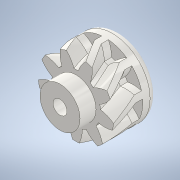
# Autodesk Inventor part: Spur Gear1
Saved by Autodesk Inventor 2022 (Build 260153070, 153G)
## iProperties
CustomPartVersion: 1
Created: 2022-01-11
Part Number: Spur Gear1
Material: Steel
Document SubType Name: Modeling
Designer: a laptop
Categories: <?xml version="1.0" encoding="UTF-16"?> <MemberInstance><Categories><FamilyTemplate><FamilyTemplateParameter ValueType="xs:double" Id="1" ObjectReferenceKey="da_z" ObjectType="kUserParameterObject"/><FamilyTemplateParameter ValueType="xs:double" Id="2" ObjectReferenceKey="da_b" ObjectType="kUserParameterObject"/><FamilyTemplateParameter ValueType="xs:double" Id="3" ObjectReferenceKey="da_beta" ObjectType="kUserParameterObject"/><FamilyTemplateParameter ValueType="xs:double" Id="4" ObjectReferenceKey="da_da" ObjectType="kUserParameterObject"/><FamilyTemplateParameter ValueType="xs:double" Id="5" ObjectReferenceKey="da_aw" ObjectType="kUserParameterObject"/><FamilyTemplateParameter ValueType="xs:string" Id="6" ObjectReferenceKey="EAIAABAAAACIAQAAAAAAAIAAAAAAAAAA" ObjectType="83910656" SubObjectId="SurfaceGeometry"/></FamilyTemplate><ParamToTemplateMap><ParamToTemplate CategoryParameter="//CategoryParameter[@InternalName='046C89C9-8512-4d59-83FE-43B91F4F132A']" TemplateParameter="1"/><ParamToTemplate CategoryParameter="//CategoryParameter[@InternalName='2552DF32-E462-4b46-AEBF-C6C7768E72AC']" TemplateParameter="2"/><ParamToTemplate CategoryParameter="//CategoryParameter[@InternalName='C9EE641D-15FC-4fae-A226-E94C4372FDD7']" TemplateParameter="3"/><ParamToTemplate><ParamToTemplate CategoryParameter="//CategoryParameter[@InternalName='00B6519A-459B-49c7-AD84-2E56D39A5744']" ConstantValue="0.510375"/></ParamToTemplate><ParamToTemplate><ParamToTemplate CategoryParameter="//CategoryParameter[@InternalName='04B31F0E-C7A6-4894-AA32-9629BEFACF47']" ConstantValue="1.000000"/></ParamToTemplate><ParamToTemplate><ParamToTemplate CategoryParameter="//CategoryParameter[@InternalName='43CBEC2E-7847-49e7-A936-2F7889FCB2D9']" ConstantValue="0.250000"/></ParamToTemplate><ParamToTemplate><ParamToTemplate CategoryParameter="//CategoryParameter[@InternalName='B1EFC894-105D-4ebd-86BF-FA20ED196853']" ConstantValue="0.302500"/></ParamToTemplate><ParamToTemplate><ParamToTemplate CategoryParameter="//CategoryParameter[@InternalName='51175063-3D10-4879-93E8-6246FE8B403D']" ConstantValue="2060000000.000000"/></ParamToTemplate><ParamToTemplate><ParamToTemplate CategoryParameter="//CategoryParameter[@InternalName='A3A52E27-4454-46a9-B0BD-C932399B70AF']" ConstantValue="0.300000"/></ParamToTemplate><ParamToTemplate><ParamToTemplate CategoryParameter="//CategoryParameter[@InternalName='91B76062-C214-41d9-B1B9-14D2AB99603D']" ConstantValue="0.080000"/></ParamToTemplate><ParamToTemplate><ParamToTemplate CategoryParameter="//CategoryParameter[@InternalName='374E806E-8B8A-4dda-A9AA-1039D6500AD2']" ConstantValue="12.500000"/></ParamToTemplate><ParamToTemplate><ParamToTemplate CategoryParameter="//CategoryParameter[@InternalName='2D373A89-B862-43d6-8D0B-0CBF12AB9F6C']" ConstantValue="0.261799"/></ParamToTemplate><ParamToTemplate CategoryParameter="//CategoryParameter[@InternalName='37777632-D6A2-4fac-9D53-DB8ACD95C989']" TemplateParameter="4"/><ParamToTemplate CategoryParameter="//CategoryParameter[@InternalName='FD1017F1-B727-4f7e-9707-0F86F1FF9423']" TemplateParameter="5"/><ParamToTemplate><ParamToTemplate CategoryParameter="//CategoryParameter[@InternalName='9E1B4470-B2D3-4ff1-B813-535BB4CDF51A']" ConstantValue="3520000.000000"/></ParamToTemplate><ParamToTemplate><ParamToTemplate CategoryParameter="//CategoryParameter[@InternalName='F8452263-BFF6-458c-9FB1-07C4B99E95CD']" ConstantValue="11400000.000000"/></ParamToTemplate><ParamToTemplate><ParamToTemplate CategoryParameter="//CategoryParameter[@InternalName='3E3BB259-FD49-497f-8171-6EBC954A3479']" ConstantValue="2.000000"/></ParamToTemplate><ParamToTemplate CategoryParameter="//CategoryParameter[@InternalName='27C3BAF2-7550-4e4b-AE2C-0DB134B7D9B7']" TemplateParameter="6"/></ParamToTemplateMap><Category DisplayName="Gear" InternalName="DC85795E-93AB-48d5-8EEE-5A27447B64BD" Mnemonic="Gear"><CategoryParameter DisplayName="z" InternalName="046C89C9-8512-4d59-83FE-43B91F4F132A" Mnemonic="z"/><CategoryParameter DisplayName="b" InternalName="2552DF32-E462-4b46-AEBF-C6C7768E72AC" Mnemonic="b"/><CategoryParameter DisplayName="||b|" InternalName="C9EE641D-15FC-4fae-A226-E94C4372FDD7" Mnemonic="beta"/><CategoryParameter DisplayName="x" InternalName="00B6519A-459B-49c7-AD84-2E56D39A5744" Mnemonic="x"/><CategoryParameter DisplayName="a*" InternalName="04B31F0E-C7A6-4894-AA32-9629BEFACF47" Mnemonic="a"/><CategoryParameter DisplayName="c*" InternalName="43CBEC2E-7847-49e7-A936-2F7889FCB2D9" Mnemonic="c"/><CategoryParameter DisplayName="r|.f|*" InternalName="B1EFC894-105D-4ebd-86BF-FA20ED196853" Mnemonic="rf"/><CategoryParameter DisplayName="E" InternalName="51175063-3D10-4879-93E8-6246FE8B403D" Mnemonic="E"/><CategoryParameter DisplayName="||m|" InternalName="A3A52E27-4454-46a9-B0BD-C932399B70AF" Mnemonic="mi"/><Category DisplayName="SpurGear" InternalName="26C5A22E-A91E-4dfd-A3B3-23CCAFAE1764" Mnemonic="SpurGear"><CategoryParameter DisplayName="m" InternalName="91B76062-C214-41d9-B1B9-14D2AB99603D" Mnemonic="m"/><CategoryParameter DisplayName="P" InternalName="374E806E-8B8A-4dda-A9AA-1039D6500AD2" Mnemonic="PP"/><CategoryParameter DisplayName="||a|" InternalName="2D373A89-B862-43d6-8D0B-0CBF12AB9F6C" Mnemonic="alpha"/><CategoryParameter DisplayName="d|.a|" InternalName="37777632-D6A2-4fac-9D53-DB8ACD95C989" Mnemonic="da"/><CategoryParameter DisplayName="a|.w|" InternalName="FD1017F1-B727-4f7e-9707-0F86F1FF9423" Mnemonic="aw"/><CategoryParameter DisplayName="||s||.Flim|" InternalName="9E1B4470-B2D3-4ff1-B813-535BB4CDF51A" Mnemonic="sFlim"/><CategoryParameter DisplayName="||s||.Hlim|" InternalName="F8452263-BFF6-458c-9FB1-07C4B99E95CD" Mnemonic="sHlim"/><CategoryParameter DisplayName="type" InternalName="3E3BB259-FD49-497f-8171-6EBC954A3479" Mnemonic="type"/><CategoryParameter DisplayName="PitchDiameter" InternalName="27C3BAF2-7550-4e4b-AE2C-0DB134B7D9B7" Mnemonic="IDS_PITCHDIAM"/></Category></Category></Categories></MemberInstance>
Mass: 1.41514 g
Surface Area: 2.76854 cm^2
Volume: 0.180272 cm^3
Density: 7.85 g/cm^3
Appearance: Steel
Author: a laptop
Autodesk Inventor part; units mm, degrees
ref_plane "YZ Plane" through (0, 0, 0) normal (1, 0, 0) x (0, 1, 0)
ref_plane "XZ Plane" through (0, 0, 0) normal (0, 1, 0) x (-1, 0, 0)
ref_plane "XY Plane" through (0, 0, 0) normal (0, 0, 1) x (1, 0, 0)
sketch "Sketch1" plane through (0, 0, 0) normal (0, 0, 1) x (1, 0, 0)
  circle A0 centre (0, 0) radius 5.1751
  dimension "d0" = 10.3501
  constraints: 1 centre point
  measures "d0" diameter of A0
extrude "Extrusion1" add sketch "Sketch1" along normal blind 3
ref_plane "Work Plane2" through (0, 0, 1.5) normal (0, 0, 1) x (1, 0, 0)
sketch "Sketch2" plane through (0, 0, 0) normal (0, 0, -1) x (-1, 0, 0)
  circle A0 centre (0, 0) radius 5.1751 projected
  circle A1 centre (0, 0) radius 3.9722
  dimension "d3" = 7.9443
  constraints: 1 centre point, 1 coincident
  measures "d3" diameter of A1
surface extrude "Pitch Diameter" sketch "Sketch2" against normal through all shown no curves A1
ref_plane "Work Plane8" through (0, 0, 0) normal (0.9396926, 0.3420201, 0) x (0, 0, 1)
ref_plane "Work Plane9" through (0, 0, 0) normal (1, 0, 0) x (0, 1, 0)
spur gear teeth "Spur Gear" teeth 9 pitch diameter 7.9443 tip diameter 10.3501 root diameter 6.7609 face width 3 helix angle 25 hand left start plane through (0, 0, 0) normal (0, 0, -1) x (-1, 0, 0)
sketch "Sketch3" plane through (0, 0, 0) normal (0, 0, -1) x (-1, 0, 0)
  spline S0 degree 6 poles (2.7691, 1.939) (2.9838, 2.1842) (3.1749, 2.4503) (3.3397, 2.7342) (3.4763, 3.0327) (3.5831, 3.3423) (3.6593, 3.6593) knots 0 0 0 0 0 0 0 1 1 1 1 1 1 1 projected
  arc A0 (3.6593, 3.6593) -> (2.9683, 4.2392) centre (0, 0) ccw projected
  spline S1 degree 6 poles (2.9683, 4.2392) (2.6694, 4.1091) (2.383, 3.9501) (2.1127, 3.7638) (1.8617, 3.5521) (1.6329, 3.3178) (1.4286, 3.0637) knots 0 0 0 0 0 0 0 1 1 1 1 1 1 1 projected
  spline S2 degree 6 poles (1.4286, 3.0637) (1.3395, 3.1053) (1.249, 3.1437) (1.1571, 3.179) (1.064, 3.2111) (0.9699, 3.2398) (0.8749, 3.2653) knots 0 0 0 0 0 0 0 1 1 1 1 1 1 1 projected
  spline S3 degree 6 poles (0.8749, 3.2653) (0.8818, 3.5912) (0.8571, 3.9178) (0.8009, 4.2412) (0.7136, 4.5577) (0.5964, 4.8636) (0.451, 5.1554) knots 0 0 0 0 0 0 0 1 1 1 1 1 1 1 projected
  arc A1 (0.451, 5.1554) -> (-0.451, 5.1554) centre (0, 0) ccw projected
  spline S4 degree 6 poles (-0.451, 5.1554) (-0.5964, 4.8636) (-0.7136, 4.5577) (-0.8009, 4.2412) (-0.8571, 3.9178) (-0.8818, 3.5912) (-0.8749, 3.2653) knots 0 0 0 0 0 0 0 1 1 1 1 1 1 1 projected
  spline S5 degree 6 poles (-0.8749, 3.2653) (-0.9699, 3.2398) (-1.064, 3.2111) (-1.1571, 3.179) (-1.249, 3.1437) (-1.3395, 3.1053) (-1.4286, 3.0637) knots 0 0 0 0 0 0 0 1 1 1 1 1 1 1 projected
  spline S6 degree 6 poles (-1.4286, 3.0637) (-1.6329, 3.3178) (-1.8617, 3.5521) (-2.1127, 3.7638) (-2.383, 3.9501) (-2.6694, 4.1091) (-2.9683, 4.2392) knots 0 0 0 0 0 0 0 1 1 1 1 1 1 1 projected
  arc A2 (-2.9683, 4.2392) -> (-3.6593, 3.6593) centre (0, 0) ccw projected
  spline S7 degree 6 poles (-3.6593, 3.6593) (-3.5831, 3.3423) (-3.4763, 3.0327) (-3.3397, 2.7342) (-3.1749, 2.4503) (-2.9838, 2.1842) (-2.7691, 1.939) knots 0 0 0 0 0 0 0 1 1 1 1 1 1 1 projected
  spline S8 degree 6 poles (-2.7691, 1.939) (-2.8255, 1.8584) (-2.8791, 1.7759) (-2.9298, 1.6915) (-2.9775, 1.6054) (-3.0222, 1.5178) (-3.0637, 1.4286) knots 0 0 0 0 0 0 0 1 1 1 1 1 1 1 projected
  spline S9 degree 6 poles (-3.0637, 1.4286) (-3.3835, 1.492) (-3.7094, 1.5244) (-4.0377, 1.5252) (-4.3646, 1.4942) (-4.6861, 1.4319) (-4.9987, 1.3394) knots 0 0 0 0 0 0 0 1 1 1 1 1 1 1 projected
  arc A3 (-4.9987, 1.3394) -> (-5.1554, 0.451) centre (0, 0) ccw projected
  spline S10 degree 6 poles (-5.1554, 0.451) (-4.8932, 0.2572) (-4.6124, 0.0887) (-4.3159, -0.0522) (-4.0071, -0.1638) (-3.6898, -0.2448) (-3.3676, -0.2946) knots 0 0 0 0 0 0 0 1 1 1 1 1 1 1 projected
  spline S11 degree 6 poles (-3.3676, -0.2946) (-3.359, -0.3926) (-3.347, -0.4902) (-3.3316, -0.5875) (-3.3129, -0.6841) (-3.2907, -0.7799) (-3.2653, -0.8749) knots 0 0 0 0 0 0 0 1 1 1 1 1 1 1 projected
  spline S12 degree 6 poles (-3.2653, -0.8749) (-3.551, -1.032) (-3.8215, -1.2166) (-4.0734, -1.4271) (-4.3039, -1.6609) (-4.5102, -1.9153) (-4.6902, -2.1871) knots 0 0 0 0 0 0 0 1 1 1 1 1 1 1 projected
  arc A4 (-4.6902, -2.1871) -> (-4.2392, -2.9683) centre (0, 0) ccw projected
  spline S13 degree 6 poles (-4.2392, -2.9683) (-3.9138, -2.9483) (-3.5903, -2.8968) (-3.2726, -2.8142) (-2.9644, -2.7012) (-2.6692, -2.5592) (-2.3903, -2.3903) knots 0 0 0 0 0 0 0 1 1 1 1 1 1 1 projected
  spline S14 degree 6 poles (-2.3903, -2.3903) (-2.3208, -2.4599) (-2.2489, -2.527) (-2.1746, -2.5916) (-2.0981, -2.6535) (-2.0195, -2.7127) (-1.939, -2.7691) knots 0 0 0 0 0 0 0 1 1 1 1 1 1 1 projected
  spline S15 degree 6 poles (-1.939, -2.7691) (-2.0568, -3.073) (-2.1454, -3.3884) (-2.2031, -3.7116) (-2.2294, -4.0388) (-2.2239, -4.3663) (-2.1871, -4.6902) knots 0 0 0 0 0 0 0 1 1 1 1 1 1 1 projected
  arc A5 (-2.1871, -4.6902) -> (-1.3394, -4.9987) centre (0, 0) ccw projected
  spline S16 degree 6 poles (-1.3394, -4.9987) (-1.103, -4.7742) (-0.8883, -4.5269) (-0.698, -4.2594) (-0.5346, -3.9747) (-0.3997, -3.6762) (-0.2946, -3.3676) knots 0 0 0 0 0 0 0 1 1 1 1 1 1 1 projected
  spline S17 degree 6 poles (-0.2946, -3.3676) (-0.1967, -3.3762) (-0.0984, -3.3813) (0, -3.383) (0.0984, -3.3813) (0.1967, -3.3762) (0.2946, -3.3676) knots 0 0 0 0 0 0 0 1 1 1 1 1 1 1 projected
  spline S18 degree 6 poles (0.2946, -3.3676) (0.3997, -3.6762) (0.5346, -3.9747) (0.698, -4.2594) (0.8883, -4.5269) (1.103, -4.7742) (1.3394, -4.9987) knots 0 0 0 0 0 0 0 1 1 1 1 1 1 1 projected
  arc A6 (1.3394, -4.9987) -> (2.1871, -4.6902) centre (0, 0) ccw projected
  spline S19 degree 6 poles (2.1871, -4.6902) (2.2239, -4.3663) (2.2294, -4.0388) (2.2031, -3.7116) (2.1454, -3.3884) (2.0568, -3.073) (1.939, -2.7691) knots 0 0 0 0 0 0 0 1 1 1 1 1 1 1 projected
  spline S20 degree 6 poles (1.939, -2.7691) (2.0195, -2.7127) (2.0981, -2.6535) (2.1746, -2.5916) (2.2489, -2.527) (2.3208, -2.4599) (2.3903, -2.3903) knots 0 0 0 0 0 0 0 1 1 1 1 1 1 1 projected
  spline S21 degree 6 poles (2.3903, -2.3903) (2.6692, -2.5592) (2.9644, -2.7012) (3.2726, -2.8142) (3.5903, -2.8968) (3.9138, -2.9483) (4.2392, -2.9683) knots 0 0 0 0 0 0 0 1 1 1 1 1 1 1 projected
  arc A7 (4.2392, -2.9683) -> (4.6902, -2.1871) centre (0, 0) ccw projected
  spline S22 degree 6 poles (4.6902, -2.1871) (4.5102, -1.9153) (4.3039, -1.6609) (4.0734, -1.4271) (3.8215, -1.2166) (3.551, -1.032) (3.2653, -0.8749) knots 0 0 0 0 0 0 0 1 1 1 1 1 1 1 projected
  spline S23 degree 6 poles (3.2653, -0.8749) (3.2907, -0.7799) (3.3129, -0.6841) (3.3316, -0.5875) (3.347, -0.4902) (3.359, -0.3926) (3.3676, -0.2946) knots 0 0 0 0 0 0 0 1 1 1 1 1 1 1 projected
  spline S24 degree 6 poles (3.3676, -0.2946) (3.6898, -0.2448) (4.0071, -0.1638) (4.3159, -0.0522) (4.6124, 0.0887) (4.8932, 0.2572) (5.1554, 0.451) knots 0 0 0 0 0 0 0 1 1 1 1 1 1 1 projected
  arc A8 (5.1554, 0.451) -> (4.9987, 1.3394) centre (0, 0) ccw projected
  spline S25 degree 6 poles (4.9987, 1.3394) (4.6861, 1.4319) (4.3646, 1.4942) (4.0377, 1.5252) (3.7094, 1.5244) (3.3835, 1.492) (3.0637, 1.4286) knots 0 0 0 0 0 0 0 1 1 1 1 1 1 1 projected
  spline S26 degree 6 poles (3.0637, 1.4286) (3.0222, 1.5178) (2.9775, 1.6054) (2.9298, 1.6915) (2.8791, 1.7759) (2.8255, 1.8584) (2.7691, 1.939) knots 0 0 0 0 0 0 0 1 1 1 1 1 1 1 projected
  circle A9 centre (0, 0) radius 0.75
  dimension "d52" = 1.5
  constraints: 1 centre point, 1 coincident, 1 horizontal alignment, 26 other
  measures "d52" diameter of A9
extrude "Extrusion2" add sketch "Sketch3" along normal blind 1
sketch "Sketch4" plane through (0, 0, -1) normal (0, 0, -1) x (-1, 0, 0)
  circle A0 centre (0, 0) radius 5.1751
  arc A1 (0.451, 5.1554) -> (-0.451, 5.1554) centre (0, 0) ccw projected
  circle A2 centre (0, 0) radius 3.075
  point P0 (0, 5.1751)
  dimension "d55" = 6.15
  constraints: 2 coincident, 1 centre point, 1 point on circle, 1 vertical alignment, 2 other
  measures "d55" diameter of A2
extrude "Extrusion3" add sketch "Sketch4" along normal blind 2
fillet "Fillet1" radius 1 1 edges at (5.1751, 0, -3)
sketch "Sketch6" plane through (0, 0, 3) normal (0, 0, 1) x (1, 0, 0)
  circle A0 centre (0, 0) radius 1.875
  dimension "d66" = 3.75
  constraints: 1 centre point, 1 coincident
  measures "d66" diameter of A0
extrude "Extrusion5" add sketch "Sketch6" along normal blind 2.2
sketch "Sketch5" plane through (0, 0, 3) normal (0, 0, 1) x (1, 0, 0)
  circle A0 centre (0, 0) radius 0.95
  dimension "d59" = 1.9
  constraints: 1 centre point, 1 coincident
  measures "d59" diameter of A0
extrude "Extrusion4" cut sketch "Sketch5" along normal blind 2.9 and the other way blind 2
equation "\"d0\" = da_da"
equation "\"d1\" = da_b"
equation "\"d3\" = da_d"
equation "\"da_da\" = 10.350115"
equation "\"da_b\" = 3"
equation "\"da_d\" = 7.944321"
body "Solid1"
body "Srf1"
